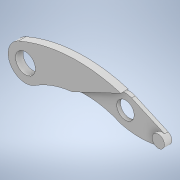
# Autodesk Inventor part: 揺動節
Saved by Autodesk Inventor 2022.2 (Build 262287000, 287)
## iProperties
Created: 2021-12-28
Part Number: 揺動節
Material: Generic
Document SubType Name: Modeling
Designer: acps
Density: 1 g/cm^3
Appearance: Default
Author: acps
Autodesk Inventor part; units mm, degrees
ref_plane "YZ Plane" through (0, 0, 0) normal (1, 0, 0) x (0, 1, 0)
ref_plane "XZ Plane" through (0, 0, 0) normal (0, 1, 0) x (-1, 0, 0)
ref_plane "XY Plane" through (0, 0, 0) normal (0, 0, 1) x (1, 0, 0)
sketch "Sketch1" plane through (0, 0, 0) normal (0, 0, 1) x (1, 0, 0)
  line L0 (62.53, 14) -> (101.4624, 16.295) construction
  circle A0 centre (62.53, 14) radius 3 construction
  circle A1 centre (62.53, 14) radius 4.025
  circle A2 centre (62.53, 14) radius 7
  arc A3 (103.4519, 21.9556) -> (59.7528, 20.4255) centre (83.5576, -34.6502) ccw
  arc A4 (99.0845, 10.7863) -> (66.3106, 8.1087) centre (85.2135, -21.3477) ccw
  circle A5 centre (101.4624, 16.295) radius 2.5 construction
  circle A6 centre (101.4624, 16.295) radius 3.525
  circle A7 centre (101.4624, 16.295) radius 6
  line L1 (0, 0) -> (182.8214, 0)
  line L2 (62.53, 14) -> (100, 0) construction
  line L3 (101.4624, 16.295) -> (118.735, -7) construction
  line L4 (118.735, -7) -> (100, 0) construction
  circle A8 centre (118.735, -7) radius 10 construction
  circle A9 centre (118.735, -7) radius 7.025 construction
  line L5 (105.7431, 20.4993) -> (125.8695, 0.0071) construction
  line L6 (96.1959, 13.4203) -> (109.9575, -11.7912) construction
  line L7 (113.0553, 13.1969) -> (119.7295, 6.4013) construction
  circle A10 centre (116.2097, 13.553) radius 2.5
  line L8 (117.2276, 15.8364) -> (103.9054, 21.7752)
  arc A11 (100.0011, 10.4757) -> (117.0189, 11.1876) centre (107.3077, 39.5723) ccw
  line L9 (101.4624, 16.295) -> (77.2023, 0.4065) construction
  circle A12 centre (77.2023, 0.4065) radius 10 construction
  line L10 (98.8989, 21.7198) -> (72.9297, 9.4478) construction
  line L11 (81.3819, 13.442) -> (101.059, 22.7406)
  dimension "d10" = 12
  dimension "d21" = 20
  dimension "d0" = 39
  dimension "d1" = 8.05
  dimension "d2" = 6
  dimension "d3" = 14
  dimension "d4" = 60
  dimension "d5" = 35
  dimension "d6" = 14
  dimension "d7" = 40
  dimension "d8" = 29
  dimension "d9" = 20
  dimension "d11" = 7.05
  dimension "d12" = 20
  dimension "d13" = 14.05
  dimension "d14" = 180
  dimension "d15" = 0.1
  dimension "d16" = 5
  dimension "d17" = 15
  dimension "d18" = 30
  dimension "d19" = 5
  dimension "d20" = 29
  dimension "d26" = 21.92
  constraints: 24 end point, 14 point on circle, 11 centre point, 9 coincident, 7 tangent, 2 point on line, 1 horizontal, 1 parallel, 22 other
  measures "d0" distance of L0.start L0.end
  measures "d1" diameter of A1
  measures "d2" diameter of A0
  measures "d3" diameter of A2
  measures "d4" radius of A3
  measures "d5" radius of A4
  measures "d6" distance from line of L1 L0.start
  measures "d7" distance of L2.start L2.end
  measures "d8" distance of L3.start L3.end
  measures "d9" distance of L3.end L2.end
  measures "d11" diameter of A6
  measures "d12" diameter of A8
  measures "d13" diameter of A9
  measures "d14" angle of L2 L4
  measures "d15" distance between parallel lines of L5 L7
  measures "d16" diameter of A10
  measures "d17" distance of A10.centre L0.end
  measures "d18" radius of A11
  measures "d19" diameter of A5
  measures "d20" distance of L3.start L9.end
  measures "d26" angle of L0 L10
extrude "Extrusion1" add sketch "Sketch1" along normal blind 3 contours A2 | A2 A3 L11 A4 | A10
extrude "Extrusion2" add sketch "Sketch1" along normal blind 1.5 contours L11 A7 A4 | A7 | L8 A10 A11 A7
body "Solid1"
